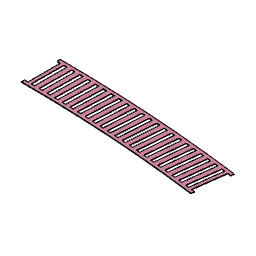
0_15m_Joch_Gebogen_Schablone_v8 (Autodesk Fusion 360 design; units mm, degrees)
Autodesk Fusion 360 part; units mm, degrees
sketch "Skizze4" plane through (0, 0, 0) normal (0, 0, 1) x (1, 0, 0)
  line L0 (0, 0) -> (0, -2516) construction
  circle A0 centre (0, -2516) radius 2516 construction
  line L1 (9.163, 13.0852) -> (9.1, -0.0147)
  line L2 (9.1, -0.0147) -> (15.1, -0.0435)
  line L3 (15.1, -0.0435) -> (15.163, 13.0563)
  line L4 (15.163, 13.0563) -> (9.163, 13.0852)
  line L5 (-3, 13.1) -> (3, 13.1)
  line L6 (3, 13.1) -> (3, 0)
  line L7 (3, 0) -> (-3, 0)
  line L8 (-3, 0) -> (-3, 13.1)
  line L9 (12.163, 13.0708) -> (12.1, -0.0291) construction
  line L10 (23.6378, 12.9913) -> (23.4998, -0.108)
  line L11 (29.4995, -0.1712) -> (29.6374, 12.9281)
  line L12 (26.6376, 12.9597) -> (26.4996, -0.1396) construction
  line L13 (29.6374, 12.9281) -> (23.6378, 12.9913)
  line L14 (23.4998, -0.108) -> (29.4995, -0.1712)
  line L15 (38.1117, 12.8146) -> (37.8988, -0.2837)
  line L16 (58.583, 12.4232) -> (52.5845, 12.5551)
  line L17 (52.2966, -0.5418) -> (58.2951, -0.6736)
  line L18 (52.5845, 12.5551) -> (52.2966, -0.5418)
  line L19 (58.2951, -0.6736) -> (58.583, 12.4232)
  line L20 (55.5837, 12.4891) -> (55.2958, -0.6077) construction
  line L21 (41.1113, 12.7658) -> (40.8984, -0.3324) construction
  line L22 (37.8988, -0.2837) -> (43.898, -0.3812)
  line L23 (43.898, -0.3812) -> (44.111, 12.7171)
  line L24 (44.111, 12.7171) -> (38.1117, 12.8146)
  line L25 (115.8597, -2.6672) -> (116.4473, 10.4196)
  line L26 (101.4731, -2.0453) -> (101.9858, 11.0447)
  line L27 (81.5243, 11.7875) -> (81.0865, -1.3052)
  line L28 (101.9858, 11.0447) -> (95.9904, 11.2795)
  line L29 (67.0555, 12.2127) -> (66.6926, -0.8823)
  line L30 (109.8657, -2.3981) -> (115.8597, -2.6672)
  line L31 (87.5209, 11.587) -> (81.5243, 11.7875)
  line L32 (66.6926, -0.8823) -> (72.6903, -1.0485)
  line L33 (70.0543, 12.1296) -> (69.6914, -0.9654) construction
  line L34 (113.4504, 10.5541) -> (112.8627, -2.5327) construction
  line L35 (81.0865, -1.3052) -> (87.0831, -1.5057)
  line L36 (72.6903, -1.0485) -> (73.0532, 12.0465)
  line L37 (84.5226, 11.6872) -> (84.0848, -1.4055) construction
  line L38 (98.9881, 11.1621) -> (98.4754, -1.9279) construction
  line L39 (95.9904, 11.2795) -> (95.4777, -1.8105)
  line L40 (110.4534, 10.6887) -> (109.8657, -2.3981)
  line L41 (95.4777, -1.8105) -> (101.4731, -2.0453)
  line L42 (116.4473, 10.4196) -> (110.4534, 10.6887)
  line L43 (73.0532, 12.0465) -> (67.0555, 12.2127)
  line L44 (87.0831, -1.5057) -> (87.5209, 11.587)
  line L45 (197.1387, 5.4068) -> (196.1021, -7.6521)
  line L46 (139.368, 9.2589) -> (138.6306, -3.8204)
  line L47 (153.8187, 8.4199) -> (153.0065, -4.6549)
  line L48 (214.5556, 3.9827) -> (213.4443, -9.0701) construction
  line L49 (173.3636, -5.9781) -> (174.2506, 7.0919)
  line L50 (171.2575, 7.295) -> (170.3704, -5.7749) construction
  line L51 (138.6306, -3.8204) -> (144.6211, -4.1581)
  line L52 (153.0065, -4.6549) -> (158.9949, -5.027)
  line L53 (200.1293, 5.1694) -> (199.0927, -7.8895) construction
  line L54 (145.3585, 8.9211) -> (139.368, 9.2589)
  line L55 (211.5664, 4.2372) -> (210.4551, -8.8156)
  line L56 (224.8012, -10.0612) -> (230.7766, -10.6044)
  line L57 (231.9626, 2.4418) -> (225.9872, 2.985)
  line L58 (124.9127, 10.0152) -> (124.2502, -3.0681)
  line L59 (182.7046, 6.4938) -> (181.7427, -6.5709)
  line L60 (167.3773, -5.5718) -> (173.3636, -5.9781)
  line L61 (217.5448, 3.7282) -> (211.5664, 4.2372)
  line L62 (210.4551, -8.8156) -> (216.4335, -9.3246)
  line L63 (228.9749, 2.7134) -> (227.7889, -10.3328) construction
  line L64 (185.6965, 6.2735) -> (184.7346, -6.7911) construction
  line L65 (130.9051, 9.7117) -> (124.9127, 10.0152)
  line L66 (130.2425, -3.3715) -> (130.9051, 9.7117)
  line L67 (202.0833, -8.1269) -> (203.1199, 4.932)
  line L68 (159.8072, 8.0478) -> (153.8187, 8.4199)
  line L69 (158.9949, -5.027) -> (159.8072, 8.0478)
  line L70 (230.7766, -10.6044) -> (231.9626, 2.4418)
  line L71 (168.2644, 7.4981) -> (167.3773, -5.5718)
  line L72 (156.813, 8.2338) -> (156.0007, -4.8409) construction
  line L73 (188.6884, 6.0532) -> (182.7046, 6.4938)
  line L74 (142.3633, 9.09) -> (141.6259, -3.9892) construction
  line L75 (187.7265, -7.0114) -> (188.6884, 6.0532)
  line L76 (127.9089, 9.8634) -> (127.2464, -3.2198) construction
  line L77 (203.1199, 4.932) -> (197.1387, 5.4068)
  line L78 (181.7427, -6.5709) -> (187.7265, -7.0114)
  line L79 (174.2506, 7.0919) -> (168.2644, 7.4981)
  line L80 (196.1021, -7.6521) -> (202.0833, -8.1269)
  line L81 (225.9872, 2.985) -> (224.8012, -10.0612)
  line L82 (144.6211, -4.1581) -> (145.3585, 8.9211)
  line L83 (216.4335, -9.3246) -> (217.5448, 3.7282)
  line L84 (124.2502, -3.0681) -> (130.2425, -3.3715)
  line L85 (0, 13.1) -> (0, 0) construction
  line L86 (243.3867, 1.3617) -> (242.126, -11.6775) construction
  line L87 (275.1684, -1.9121) -> (269.2033, -1.2663)
  line L88 (288.0686, -16.5438) -> (282.1073, -15.8639)
  line L89 (286.5723, -3.1882) -> (285.0879, -16.2038) construction
  line L90 (269.2033, -1.2663) -> (267.7934, -14.2902)
  line L91 (246.3728, 1.073) -> (240.4006, 1.6504)
  line L92 (282.1073, -15.8639) -> (283.5916, -2.8483)
  line L93 (245.1121, -11.9662) -> (246.3728, 1.073)
  line L94 (253.4708, -12.7985) -> (259.4396, -13.4101)
  line L95 (289.553, -3.5281) -> (288.0686, -16.5438)
  line L96 (240.4006, 1.6504) -> (239.1399, -11.3888)
  line L97 (273.7586, -14.936) -> (275.1684, -1.9121)
  line L98 (259.4396, -13.4101) -> (260.7749, -0.3784)
  line L99 (239.1399, -11.3888) -> (245.1121, -11.9662)
  line L100 (254.8061, 0.2332) -> (253.4708, -12.7985)
  line L101 (283.5916, -2.8483) -> (289.553, -3.5281)
  line L102 (260.7749, -0.3784) -> (254.8061, 0.2332)
  line L103 (272.1859, -1.5892) -> (270.776, -14.6131) construction
  line L104 (257.7905, -0.0726) -> (256.4552, -13.1043) construction
  line L105 (267.7934, -14.2902) -> (273.7586, -14.936)
  line L106 (315.3166, -6.6331) -> (313.6833, -19.6309) construction
  line L107 (318.2932, -7.0071) -> (312.34, -6.2591)
  line L108 (322.8097, -20.7928) -> (328.7592, -21.5697)
  line L109 (324.506, -7.8031) -> (322.8097, -20.7928)
  line L110 (316.6599, -20.0049) -> (318.2932, -7.0071)
  line L111 (312.34, -6.2591) -> (310.7067, -19.2569)
  line L112 (303.9281, -5.2265) -> (297.9707, -4.5125)
  line L113 (297.9707, -4.5125) -> (296.4118, -17.5195)
  line L114 (296.4118, -17.5195) -> (302.3692, -18.2334)
  line L115 (300.9494, -4.8695) -> (299.3905, -17.8764) construction
  line L116 (327.4807, -8.1916) -> (325.7844, -21.1813) construction
  line L117 (302.3692, -18.2334) -> (303.9281, -5.2265)
  line L118 (330.4554, -8.58) -> (324.506, -7.8031)
  line L119 (328.7592, -21.5697) -> (330.4554, -8.58)
  line L120 (310.7067, -19.2569) -> (316.6599, -20.0049)
  point P0 (12.1, -0.0291)
  point P1 (26.4996, -0.1396)
  point P2 (55.2958, -0.6077)
  point P3 (40.8984, -0.3324)
  point P4 (112.8627, -2.5327)
  point P5 (98.4754, -1.9279)
  point P6 (84.0848, -1.4055)
  point P7 (69.6914, -0.9654)
  point P8 (170.3704, -5.7749)
  point P9 (156.0007, -4.8409)
  point P10 (199.0927, -7.8895)
  point P11 (184.7346, -6.7911)
  point P12 (213.4443, -9.0701)
  point P13 (227.7889, -10.3328)
  point P14 (141.6259, -3.9892)
  point P15 (127.2464, -3.2198)
  point P16 (256.4552, -13.1043)
  point P17 (242.126, -11.6775)
  point P18 (285.0879, -16.2038)
  point P19 (270.776, -14.6131)
  point P20 (313.6833, -19.6309)
  point P21 (325.7844, -21.1813)
  point P22 (299.3905, -17.8764)
  dimension "d197" = 2516
  dimension "d198" = 6
  dimension "d199" = 13.1
  dimension "d200" = 6
  dimension "d201" = 13.1
  dimension "d202" = 6
  dimension "d203" = 13.1
  dimension "d204" = 6
  dimension "d205" = 13.1
  dimension "d206" = 6
  dimension "d207" = 13.1
  dimension "d208" = 6
  dimension "d209" = 13.1
  dimension "d210" = 6
  dimension "d211" = 13.1
  dimension "d212" = 6
  dimension "d213" = 13.1
  dimension "d214" = 6
  dimension "d215" = 13.1
  dimension "d216" = 6
  dimension "d217" = 13.1
  dimension "d218" = 6
  dimension "d219" = 13.1
  dimension "d220" = 6
  dimension "d221" = 13.1
  dimension "d222" = 6
  dimension "d223" = 13.1
  dimension "d224" = 6
  dimension "d225" = 13.1
  dimension "d226" = 6
  dimension "d227" = 13.1
  dimension "d228" = 6
  dimension "d229" = 13.1
  dimension "d230" = 6
  dimension "d231" = 13.1
  dimension "d232" = 12.1
  dimension "d233" = 14.4
  dimension "d234" = 14.4
  dimension "d235" = 14.4
  dimension "d236" = 14.4
  dimension "d237" = 14.4
  dimension "d238" = 14.4
  dimension "d239" = 14.4
  dimension "d240" = 6
  dimension "d241" = 13.1
  dimension "d242" = 6
  dimension "d243" = 13.1
  dimension "d244" = 6
  dimension "d245" = 13.1
  dimension "d246" = 6
  dimension "d247" = 13.1
  dimension "d248" = 6
  dimension "d249" = 13.1
  dimension "d250" = 6
  dimension "d251" = 13.1
  dimension "d252" = 6
  dimension "d253" = 13.1
  dimension "d254" = 14.4
  dimension "d255" = 14.4
  dimension "d256" = 14.4
  dimension "d257" = 14.4
  dimension "d258" = 14.4
  dimension "d259" = 14.4
  dimension "d260" = 14.4
  dimension "d261" = 14.4
  dimension "d262" = 14.4
  dimension "d263" = 14.4
  dimension "d264" = 14.4
  dimension "d265" = 14.4
  dimension "d266" = 14.4
  dimension "d267" = 14.4
  dimension "d268" = 12.2
  dimension "d269" = 7.4
  constraint coincident L0.start L85.end
  constraint vertical L0
  constraint coincident L0.end A0.centre
  constraint coincident L0.start A0
  constraint perpendicular L1 L2
  constraint parallel L1 L3
  constraint parallel L2 L4
  constraint midpoint L2 P0
  constraint horizontal L5
  constraint vertical L6
  constraint horizontal L7
  constraint vertical L8
  constraint midpoint L0.start L7
  constraint midpoint L4 L9.start
  constraint coincident P0 L9.end
  constraint perpendicular L10 L14
  constraint parallel L10 L11
  constraint parallel L13 L14
  constraint midpoint P1 L14
  constraint midpoint L12.start L13
  constraint coincident P1 L12.end
  constraint perpendicular L15 L22
  constraint parallel L15 L23
  constraint parallel L22 L24
  constraint midpoint P3 L22
  constraint midpoint L21.start L24
  constraint coincident P3 L21.end
  constraint perpendicular L17 L18
  constraint parallel L18 L19
  constraint parallel L16 L17
  constraint midpoint P2 L17
  constraint midpoint L20.start L16
  constraint coincident P2 L20.end
  constraint perpendicular L29 L32
  constraint parallel L29 L36
  constraint parallel L32 L43
  constraint midpoint P7 L32
  constraint midpoint L33.start L43
  constraint coincident P7 L33.end
  constraint perpendicular L27 L35
  constraint parallel L27 L44
  constraint parallel L31 L35
  constraint midpoint P6 L35
  constraint midpoint L37.start L31
  constraint coincident P6 L37.end
  constraint perpendicular L39 L41
  constraint parallel L26 L39
  constraint parallel L28 L41
  constraint midpoint P5 L41
  constraint midpoint L38.start L28
  constraint coincident P5 L38.end
  constraint perpendicular L30 L40
  constraint parallel L25 L40
  constraint parallel L30 L42
  constraint midpoint P4 L30
  constraint midpoint L34.start L42
  constraint coincident P4 L34.end
  constraint perpendicular L58 L84
  constraint parallel L58 L66
  constraint parallel L65 L84
  constraint midpoint P15 L84
  constraint midpoint L76.start L65
  constraint coincident P15 L76.end
  constraint perpendicular L46 L51
  constraint parallel L46 L82
  constraint parallel L51 L54
  constraint midpoint P14 L51
  constraint midpoint L74.start L54
  constraint coincident P14 L74.end
  constraint perpendicular L47 L52
  constraint parallel L47 L69
  constraint parallel L52 L68
  constraint midpoint P9 L52
  constraint midpoint L72.start L68
  constraint coincident P9 L72.end
  constraint perpendicular L60 L71
  constraint parallel L49 L71
  constraint parallel L60 L79
  constraint midpoint P8 L60
  constraint midpoint L50.start L79
  constraint coincident P8 L50.end
  constraint perpendicular L59 L78
  constraint parallel L59 L75
  constraint parallel L73 L78
  constraint midpoint P11 L78
  constraint midpoint L64.start L73
  constraint coincident P11 L64.end
  constraint perpendicular L45 L80
  constraint parallel L45 L67
  constraint parallel L77 L80
  constraint midpoint P10 L80
  constraint midpoint L53.start L77
  constraint coincident P10 L53.end
  constraint perpendicular L55 L62
  constraint parallel L55 L83
  constraint parallel L61 L62
  constraint midpoint P12 L62
  constraint midpoint L48.start L61
  constraint coincident P12 L48.end
  constraint perpendicular L56 L81
  constraint parallel L70 L81
  constraint parallel L56 L57
  constraint midpoint P13 L56
  constraint midpoint L63.start L57
  constraint coincident P13 L63.end
  constraint midpoint L5 L85.start
  constraint coincident A0 P0
  constraint coincident A0 P1
  constraint coincident A0 P3
  constraint coincident A0 P2
  constraint coincident A0 P7
  constraint coincident A0 P6
  constraint coincident A0 P5
  constraint coincident A0 P4
  constraint tangent A0 L2
  constraint tangent A0 L14
  constraint tangent A0 L22
  constraint tangent A0 L17
  constraint tangent A0 L32
  constraint tangent A0 L35
  constraint tangent A0 L41
  constraint tangent A0 L30
  constraint coincident A0 P15
  constraint coincident A0 P14
  constraint coincident A0 P9
  constraint coincident A0 P8
  constraint perpendicular L96 L99
  constraint parallel L93 L96
  constraint parallel L91 L99
  constraint midpoint P17 L99
  constraint midpoint L86.start L91
  constraint coincident P17 L86.end
  constraint perpendicular L94 L100
  constraint parallel L98 L100
  constraint parallel L94 L102
  constraint midpoint P16 L94
  constraint midpoint L104.start L102
  constraint coincident P16 L104.end
  constraint perpendicular L90 L105
  constraint parallel L90 L97
  constraint parallel L87 L105
  constraint midpoint P19 L105
  constraint midpoint L103.start L87
  constraint coincident P19 L103.end
  constraint perpendicular L88 L95
  constraint parallel L92 L95
  constraint parallel L88 L101
  constraint midpoint P18 L88
  constraint midpoint L89.start L101
  constraint coincident P18 L89.end
  constraint perpendicular L113 L114
  constraint parallel L113 L117
  constraint parallel L112 L114
  constraint midpoint P22 L114
  constraint midpoint L115.start L112
  constraint coincident P22 L115.end
  constraint perpendicular L111 L120
  constraint parallel L110 L111
  constraint parallel L107 L120
  constraint midpoint P20 L120
  constraint midpoint L106.start L107
  constraint coincident P20 L106.end
  constraint perpendicular L108 L109
  constraint parallel L109 L119
  constraint parallel L108 L118
  constraint midpoint P21 L108
  constraint midpoint L116.start L118
  constraint coincident P21 L116.end
  constraint coincident A0 P11
  constraint coincident A0 P10
  constraint coincident A0 P12
  constraint coincident A0 P13
  constraint tangent A0 L84
  constraint tangent A0 L51
  constraint tangent A0 L52
  constraint tangent A0 L60
  constraint tangent A0 L78
  constraint tangent A0 L80
  constraint tangent A0 L62
  constraint tangent A0 L56
  constraint coincident A0 P17
  constraint coincident A0 P16
  constraint coincident A0 P19
  constraint coincident A0 P18
  constraint coincident A0 P22
  constraint coincident A0 P20
  constraint coincident A0 P21
  constraint tangent A0 L99
  constraint tangent A0 L94
  constraint tangent A0 L105
  constraint tangent A0 L88
  constraint tangent A0 L114
  constraint tangent A0 L120
  constraint tangent A0 L108
  measures "d197" distance of L0.start L0.end
  measures "d198" distance of L1 L3
  measures "d199" distance of L2 L4
  measures "d200" distance of L6 L8
  measures "d201" distance of L5 L7
  measures "d202" distance of L10 L11
  measures "d203" distance of L13 L14
  measures "d204" distance of L15 L23
  measures "d205" distance of L22 L24
  measures "d206" distance of L18 L19
  measures "d207" distance of L16 L17
  measures "d208" distance of L29 L36
  measures "d209" distance of L32 L43
  measures "d210" distance of L27 L44
  measures "d211" distance of L31 L35
  measures "d212" distance of L26 L39
  measures "d213" distance of L28 L41
  measures "d214" distance of L25 L40
  measures "d215" distance of L30 L42
  measures "d216" distance of L58 L66
  measures "d217" distance of L65 L84
  measures "d218" distance of L46 L82
  measures "d219" distance of L51 L54
  measures "d220" distance of L47 L69
  measures "d221" distance of L52 L68
  measures "d222" distance of L49 L71
  measures "d223" distance of L60 L79
  measures "d224" distance of L59 L75
  measures "d225" distance of L73 L78
  measures "d226" distance of L45 L67
  measures "d227" distance of L77 L80
  measures "d228" distance of L55 L83
  measures "d229" distance of L61 L62
  measures "d230" distance of L70 L81
  measures "d231" distance of L56 L57
  measures "d232" distance of P0 L85
  measures "d233" distance of L9 P1
  measures "d234" distance of L12 P3
  measures "d235" distance of P2 L21
  measures "d236" distance of L20 P7
  measures "d237" distance of P6 L33
  measures "d238" distance of P5 L37
  measures "d239" distance of P4 L38
  measures "d240" distance of L93 L96
  measures "d241" distance of L91 L99
  measures "d242" distance of L98 L100
  measures "d243" distance of L94 L102
  measures "d244" distance of L90 L97
  measures "d245" distance of L87 L105
  measures "d246" distance of L92 L95
  measures "d247" distance of L88 L101
  measures "d248" distance of L113 L117
  measures "d249" distance of L112 L114
  measures "d250" distance of L110 L111
  measures "d251" distance of L107 L120
  measures "d252" distance of L109 L119
  measures "d253" distance of L108 L118
  measures "d254" distance of L34 P15
  measures "d255" distance of P14 L76
  measures "d256" distance of P9 L74
  measures "d257" distance of P8 L72
  measures "d258" distance of P11 L50
  measures "d259" distance of P10 L64
  measures "d260" distance of P12 L53
  measures "d261" distance of P13 L48
  measures "d262" distance of L63 P17
  measures "d263" distance of P16 L86
  measures "d264" distance of P19 L104
  measures "d265" distance of P18 L103
  measures "d266" distance of L89 P22
  measures "d267" distance of P20 L115
  measures "d268" distance of P21 L106
extrude "Extrusion1" add sketch "Skizze4" along normal blind 3 makes body 1 at (27.5456, 4.2163, 0) makes body 2 at (83.2313, 2.9922, 0) makes body 3 at (140.8732, 0.4268, 0) makes body 4 at (198.4414, -3.4574, 0) makes body 5 at (258.3402, -4.5184, 0) makes body 6 at (313.2355, -15.1736, 0) makes body 7 at (298.9172, -13.4218, 0) makes body 8 at (243.5416, -7.4274, 0) makes body 9 at (184.0579, -2.3628, 0) makes body 10 at (126.4685, 1.1919, 0) makes body 11 at (68.8128, 3.4273, 0) makes body 12 at (13.121, 4.3327, 0) makes body 13 at (39.9695, 4.0499, 0) makes body 14 at (97.647, 2.4746, 0) makes body 15 at (155.2734, -0.4207, 0) makes body 16 at (212.8183, -4.6343, 0) makes body 17 at (270.2518, -10.1642, 0) makes body 18 at (327.9069, -12.6509, 0) makes body 19 at (287.0711, -7.6401, 0) makes body 20 at (229.1801, -6.0746, 0) makes body 21 at (169.6684, -1.3506, 0) makes body 22 at (112.2555, 6.2367, 0) makes body 23 at (54.392, 3.7799, 0) makes body 24 at (-1, 4.3667, 0)
move_face "Flächen versetzen1" offset 45.1 24 faces at (300.3834, -17.9954, 2) (241.1307, -11.5813, 1) (183.7373, -6.7177, 1) (128.2451, -3.2704, 2) (83.0853, -1.372, 1) (25.4997, -0.129, 1) (255.4604, -13.0024, 1) (314.6755, -19.7556, 2) (198.0958, -7.8104, 1) (140.6274, -3.9329, 1) (68.6918, -0.9377, 1) (13.1, -0.0339, 2) (39.8985, -0.3162, 1) (97.4761, -1.8887, 2) (155.0026, -4.7789, 1) (212.4479, -8.9853, 1) (269.7818, -14.5055, 1) (324.7929, -21.0518, 1) (286.0815, -16.3171, 1) (226.793, -10.2422, 1) (169.3727, -5.7072, 1) (111.8637, -2.4878, 1) (54.2961, -0.5857, 1) (1, 0, 1) on bodies 1 2 3 4 5 6 7 8 9 10 11 12 13 14 15 16 17 18 19 20 21 22 23 24
sketch "Skizze5" plane through (0, 0, 0) normal (0, 0, 1) x (1, 0, 0)
  line L0 (-3, 13.1) -> (-3, -45.1)
  line L1 (322.9194, -66.29) -> (330.4554, -8.58)
  line L2 (-3, 13.1) -> (-3, 18.7667)
  line L3 (-3, -45.1) -> (-3, -50.7667)
  line L4 (330.4554, -8.58) -> (331.1892, -2.9611)
  line L5 (322.9194, -66.29) -> (322.1856, -71.909)
  arc A0 (331.1892, -2.9611) -> (-3, 18.7667) centre (-3, -2562.142) ccw
  arc A1 (322.1856, -71.909) -> (-3, -50.7667) centre (-3, -2562.142) ccw
  line L6 (-3, 18.7667) -> (-30, 18.7667)
  line L7 (-3, -50.7667) -> (-34, -50.7667)
  dimension "d273" = 5.6667
  dimension "d274" = 5.6667
  dimension "d275" = 5.6667
  dimension "d276" = 5.6667
  constraint coincident L0.start L2.start
  constraint coincident L0.end L3.start
  constraint coincident L1.end L4.start
  constraint coincident L1.start L5.start
  constraint parallel L0 L2
  constraint parallel L0 L3
  constraint parallel L1 L5
  constraint parallel L1 L4
  constraint perpendicular L2 L6
  constraint tangent A0 L6
  constraint perpendicular L3 L7
  constraint tangent A1 L7
  measures "d273" distance of L0.start L2.end
  measures "d274" distance of L0.end L3.end
  measures "d275" distance of L1.end L4.end
  measures "d276" distance of L1.start L5.end
extrude "Extrusion2" add sketch "Skizze5" along normal blind 1 separate body makes body 25
combine "Kombinieren1" operation cut target body 25 tool bodies 18 6 7 19 17 5 8 20 16 4 9 21 15 3 10 22 14 2 11 23 13 1 12 24 keep tools
sketch "Skizze8" plane through (0, 0, 1) normal (0, 0, 1) x (-1, 0, 0)
  line L0 (-3, 45.1) -> (3, 45.1)
  line L1 (3, 45.1) -> (3, 50.7667)
  arc A0 (-322.1856, 71.909) -> (3, 50.7667) centre (3, 2562.142) ccw
  line L2 (-322.1856, 71.909) -> (-322.9194, 66.29)
  line L3 (-322.9194, 66.29) -> (-316.9699, 65.5131)
  line L4 (-316.9699, 65.5131) -> (-324.506, 7.8031)
  line L5 (-324.506, 7.8031) -> (-330.4554, 8.58)
  line L6 (-330.4554, 8.58) -> (-331.1892, 2.9611)
  arc A1 (-331.1892, 2.9611) -> (3, -18.7667) centre (3, 2562.142) ccw
  line L7 (3, -18.7667) -> (3, -13.1)
  line L8 (3, -13.1) -> (-3, -13.1)
  line L9 (-3, -13.1) -> (-3, 45.1)
  line L10 (-15.163, -13.0563) -> (-14.8831, 45.143)
  line L11 (-14.8831, 45.143) -> (-8.8831, 45.1141)
  line L12 (-8.8831, 45.1141) -> (-9.163, -13.0852)
  line L13 (-9.163, -13.0852) -> (-15.163, -13.0563)
  line L14 (-23.0248, 45.2055) -> (-23.6378, -12.9913)
  line L15 (-23.6378, -12.9913) -> (-29.6374, -12.9281)
  line L16 (-29.6374, -12.9281) -> (-29.0245, 45.2687)
  line L17 (-29.0245, 45.2687) -> (-23.0248, 45.2055)
  line L18 (-44.111, -12.7171) -> (-43.1649, 45.4752)
  line L19 (-43.1649, 45.4752) -> (-37.1657, 45.3777)
  line L20 (-37.1657, 45.3777) -> (-38.1117, -12.8146)
  line L21 (-38.1117, -12.8146) -> (-44.111, -12.7171)
  line L22 (-57.3039, 45.7628) -> (-51.3054, 45.6309)
  line L23 (-51.3054, 45.6309) -> (-52.5845, -12.5551)
  line L24 (-52.5845, -12.5551) -> (-58.583, -12.4232)
  line L25 (-58.583, -12.4232) -> (-57.3039, 45.7628)
  line L26 (-73.0532, -12.0465) -> (-71.441, 46.1312)
  line L27 (-71.441, 46.1312) -> (-65.4433, 45.965)
  line L28 (-65.4433, 45.965) -> (-67.0555, -12.2127)
  line L29 (-67.0555, -12.2127) -> (-73.0532, -12.0465)
  line L30 (-85.5758, 46.5805) -> (-79.5792, 46.38)
  line L31 (-79.5792, 46.38) -> (-81.5243, -11.7875)
  line L32 (-81.5243, -11.7875) -> (-87.5209, -11.587)
  line L33 (-87.5209, -11.587) -> (-85.5758, 46.5805)
  line L34 (-93.7124, 46.8759) -> (-95.9904, -11.2795)
  line L35 (-95.9904, -11.2795) -> (-101.9858, -11.0447)
  line L36 (-101.9858, -11.0447) -> (-99.7078, 47.1107)
  line L37 (-99.7078, 47.1107) -> (-93.7124, 46.8759)
  line L38 (-116.4473, -10.4196) -> (-113.8366, 47.7218)
  line L39 (-113.8366, 47.7218) -> (-107.8426, 47.4527)
  line L40 (-107.8426, 47.4527) -> (-110.4534, -10.6887)
  line L41 (-110.4534, -10.6887) -> (-116.4473, -10.4196)
  line L42 (-121.9693, 48.1104) -> (-124.9127, -10.0152)
  line L43 (-124.9127, -10.0152) -> (-130.9051, -9.7117)
  line L44 (-130.9051, -9.7117) -> (-127.9616, 48.4138)
  line L45 (-127.9616, 48.4138) -> (-121.9693, 48.1104)
  line L46 (-142.0824, 49.1866) -> (-136.0919, 48.8488)
  line L47 (-136.0919, 48.8488) -> (-139.368, -9.2589)
  line L48 (-139.368, -9.2589) -> (-145.3585, -8.9211)
  line L49 (-145.3585, -8.9211) -> (-142.0824, 49.1866)
  line L50 (-156.1986, 50.0402) -> (-150.2101, 49.6682)
  line L51 (-150.2101, 49.6682) -> (-153.8187, -8.4199)
  line L52 (-153.8187, -8.4199) -> (-159.8072, -8.0478)
  line L53 (-159.8072, -8.0478) -> (-156.1986, 50.0402)
  line L54 (-174.2506, -7.0919) -> (-170.3096, 50.9746)
  line L55 (-170.3096, 50.9746) -> (-164.3234, 50.5683)
  line L56 (-164.3234, 50.5683) -> (-168.2644, -7.4981)
  line L57 (-168.2644, -7.4981) -> (-174.2506, -7.0919)
  line L58 (-178.4313, 51.5491) -> (-182.7046, -6.4938)
  line L59 (-182.7046, -6.4938) -> (-188.6884, -6.0532)
  line L60 (-188.6884, -6.0532) -> (-184.4151, 51.9897)
  line L61 (-184.4151, 51.9897) -> (-178.4313, 51.5491)
  line L62 (-192.5333, 52.6107) -> (-197.1387, -5.4068)
  line L63 (-197.1387, -5.4068) -> (-203.1199, -4.932)
  line L64 (-203.1199, -4.932) -> (-198.5145, 53.0855)
  line L65 (-198.5145, 53.0855) -> (-192.5333, 52.6107)
  line L66 (-212.6074, 54.262) -> (-206.629, 53.753)
  line L67 (-206.629, 53.753) -> (-211.5664, -4.2372)
  line L68 (-211.5664, -4.2372) -> (-217.5448, -3.7282)
  line L69 (-217.5448, -3.7282) -> (-212.6074, 54.262)
  line L70 (-225.9872, -2.985) -> (-231.9626, -2.4418)
  line L71 (-231.9626, -2.4418) -> (-226.6934, 55.5192)
  line L72 (-226.6934, 55.5192) -> (-220.718, 54.9759)
  line L73 (-220.718, 54.9759) -> (-225.9872, -2.985)
  line L74 (-234.7997, 56.2795) -> (-240.4006, -1.6504)
  line L75 (-240.4006, -1.6504) -> (-246.3728, -1.073)
  line L76 (-246.3728, -1.073) -> (-240.7719, 56.8569)
  line L77 (-240.7719, 56.8569) -> (-234.7997, 56.2795)
  line L78 (-260.7749, 0.3784) -> (-254.8425, 58.2752)
  line L79 (-254.8425, 58.2752) -> (-248.8738, 57.6636)
  line L80 (-248.8738, 57.6636) -> (-254.8061, -0.2332)
  line L81 (-254.8061, -0.2332) -> (-260.7749, 0.3784)
  line L82 (-262.9397, 59.1283) -> (-269.2033, 1.2663)
  line L83 (-269.2033, 1.2663) -> (-275.1684, 1.9121)
  line L84 (-275.1684, 1.9121) -> (-268.9048, 59.774)
  line L85 (-268.9048, 59.774) -> (-262.9397, 59.1283)
  line L86 (-283.5916, 2.8483) -> (-289.553, 3.5281)
  line L87 (-289.553, 3.5281) -> (-282.9583, 61.3533)
  line L88 (-282.9583, 61.3533) -> (-276.9969, 60.6734)
  line L89 (-276.9969, 60.6734) -> (-283.5916, 2.8483)
  line L90 (-297.0025, 63.013) -> (-291.0451, 62.299)
  line L91 (-291.0451, 62.299) -> (-297.9707, 4.5125)
  line L92 (-297.9707, 4.5125) -> (-303.9281, 5.2265)
  line L93 (-303.9281, 5.2265) -> (-297.0025, 63.013)
  line L94 (-305.0838, 64.005) -> (-312.34, 6.2591)
  line L95 (-312.34, 6.2591) -> (-318.2932, 7.0071)
  line L96 (-318.2932, 7.0071) -> (-311.037, 64.753)
  line L97 (-311.037, 64.753) -> (-305.0838, 64.005)
  line L98 (-3, -13.1) -> (-3, 45.1)
  line L99 (-8.8831, 45.1141) -> (-9.163, -13.0852)
  line L100 (-15.163, -13.0563) -> (-14.8831, 45.143)
  line L101 (-23.0248, 45.2055) -> (-23.6378, -12.9913)
  line L102 (-29.6374, -12.9281) -> (-29.0245, 45.2687)
  line L103 (-316.9699, 65.5131) -> (-324.506, 7.8031)
  line L104 (-318.2932, 7.0071) -> (-311.037, 64.753)
  line L105 (-305.0838, 64.005) -> (-312.34, 6.2591)
  line L106 (-303.9281, 5.2265) -> (-297.0025, 63.013)
  line L107 (-291.0451, 62.299) -> (-297.9707, 4.5125)
  line L108 (-3, 16) -> (7, 16)
  arc A2 (-320.7379, 36.6581) -> (-3, 16) centre (-3, 2469.858) ccw
  circle A3 centre (-3, 16) radius 1
  circle A4 centre (-9.0231, 16.0145) radius 1
  circle A5 centre (-15.023, 16.0433) radius 1
  circle A6 centre (-23.3313, 16.1071) radius 1
  point P0 (-3, 16)
  point P1 (-9.0231, 16.0145)
  point P2 (-15.023, 16.0433)
  point P3 (-23.3313, 16.1071)
  dimension "d502" = 10
  dimension "d503" = 2
  dimension "d504" = 2
  dimension "d506" = 2
  dimension "d507" = 2
  constraint midpoint L98 P0
  constraint perpendicular L98 L108
  constraint tangent L108 A2
  constraint midpoint L103 A2.start
  constraint coincident P0 L108.start
  constraint midpoint L12 P1
  constraint midpoint L10 P2
  constraint midpoint L14 P3
  constraint coincident P1 A4.centre
  constraint coincident P2 A5.centre
  constraint coincident P3 A6.centre
  measures "d502" distance of P0 L108.end
  measures "d503" diameter of A3
  measures "d504" diameter of A4
  measures "d506" diameter of A5
  measures "d507" diameter of A6
hidden bodies 1 2 3 4 5 6 7 8 9 10 11 12 13 14 15 16 17 18 19 20 21 22 23 24
equation "Schwellen_Länge = 58 mm + 0.2 mm"
equation "Schwellen_Breite = 5.8 mm + 0.2 mm"
equation "Bogen_Radius = 2500 mm"
equation "Spurweite = 32 mm"
equation "d197 = Bogen_Radius + ( Spurweite / 2 )"
equation "d198 = Schwellen_Breite"
equation "d199 = ( Schwellen_Länge / 2 ) - ( Spurweite / 2 )"
equation "d200 = Schwellen_Breite"
equation "d201 = ( Schwellen_Länge / 2 ) - ( Spurweite / 2 )"
equation "d202 = Schwellen_Breite"
equation "d203 = ( Schwellen_Länge / 2 ) - ( Spurweite / 2 )"
equation "d204 = Schwellen_Breite"
equation "d205 = ( Schwellen_Länge / 2 ) - ( Spurweite / 2 )"
equation "d206 = Schwellen_Breite"
equation "d207 = ( Schwellen_Länge / 2 ) - ( Spurweite / 2 )"
equation "d208 = Schwellen_Breite"
equation "d209 = ( Schwellen_Länge / 2 ) - ( Spurweite / 2 )"
equation "d210 = Schwellen_Breite"
equation "d211 = ( Schwellen_Länge / 2 ) - ( Spurweite / 2 )"
equation "d212 = Schwellen_Breite"
equation "d213 = ( Schwellen_Länge / 2 ) - ( Spurweite / 2 )"
equation "d214 = Schwellen_Breite"
equation "d215 = ( Schwellen_Länge / 2 ) - ( Spurweite / 2 )"
equation "d216 = Schwellen_Breite"
equation "d217 = ( Schwellen_Länge / 2 ) - ( Spurweite / 2 )"
equation "d218 = Schwellen_Breite"
equation "d219 = ( Schwellen_Länge / 2 ) - ( Spurweite / 2 )"
equation "d220 = Schwellen_Breite"
equation "d221 = ( Schwellen_Länge / 2 ) - ( Spurweite / 2 )"
equation "d222 = Schwellen_Breite"
equation "d223 = ( Schwellen_Länge / 2 ) - ( Spurweite / 2 )"
equation "d224 = Schwellen_Breite"
equation "d225 = ( Schwellen_Länge / 2 ) - ( Spurweite / 2 )"
equation "d226 = Schwellen_Breite"
equation "d227 = ( Schwellen_Länge / 2 ) - ( Spurweite / 2 )"
equation "d228 = Schwellen_Breite"
equation "d229 = ( Schwellen_Länge / 2 ) - ( Spurweite / 2 )"
equation "d230 = Schwellen_Breite"
equation "d231 = ( Schwellen_Länge / 2 ) - ( Spurweite / 2 )"
equation "d232 = Schwellen_Abstand_Anfang"
equation "d233 = Schwellen_Abstand_Mitte"
equation "d234 = Schwellen_Abstand_Mitte"
equation "d235 = Schwellen_Abstand_Mitte"
equation "d236 = Schwellen_Abstand_Mitte"
equation "d237 = Schwellen_Abstand_Mitte"
equation "d238 = Schwellen_Abstand_Mitte"
equation "d239 = Schwellen_Abstand_Mitte"
equation "d240 = Schwellen_Breite"
equation "d241 = ( Schwellen_Länge / 2 ) - ( Spurweite / 2 )"
equation "d242 = Schwellen_Breite"
equation "d243 = ( Schwellen_Länge / 2 ) - ( Spurweite / 2 )"
equation "d244 = Schwellen_Breite"
equation "d245 = ( Schwellen_Länge / 2 ) - ( Spurweite / 2 )"
equation "d246 = Schwellen_Breite"
equation "d247 = ( Schwellen_Länge / 2 ) - ( Spurweite / 2 )"
equation "d248 = Schwellen_Breite"
equation "d249 = ( Schwellen_Länge / 2 ) - ( Spurweite / 2 )"
equation "d250 = Schwellen_Breite"
equation "d251 = ( Schwellen_Länge / 2 ) - ( Spurweite / 2 )"
equation "d252 = Schwellen_Breite"
equation "d253 = ( Schwellen_Länge / 2 ) - ( Spurweite / 2 )"
equation "d254 = Schwellen_Abstand_Mitte"
equation "d255 = Schwellen_Abstand_Mitte"
equation "d256 = Schwellen_Abstand_Mitte"
equation "d257 = Schwellen_Abstand_Mitte"
equation "d258 = Schwellen_Abstand_Mitte"
equation "d259 = Schwellen_Abstand_Mitte"
equation "d260 = Schwellen_Abstand_Mitte"
equation "d261 = Schwellen_Abstand_Mitte"
equation "d262 = Schwellen_Abstand_Mitte"
equation "d263 = Schwellen_Abstand_Mitte"
equation "d264 = Schwellen_Abstand_Mitte"
equation "d265 = Schwellen_Abstand_Mitte"
equation "d266 = Schwellen_Abstand_Mitte"
equation "d267 = Schwellen_Abstand_Mitte"
equation "d268 = Schwellen_Abstand_Ende"
equation "d272 = ( Schwellen_Länge / 2 ) + ( Spurweite / 2 )"
equation "d273 = ( Trassenbrett_Breite / Schwellen_Breite / 2 ) * 1 mm"
equation "d274 = d273"
equation "d275 = d273"
equation "d276 = d273"
equation "Schwellen_Abstand_Anfang = 12.1 mm"
equation "Schwellen_Abstand_Mitte = 14.4 mm"
equation "Schwellen_Abstand_Ende = 12.2 mm"
equation "Trassenbrett_Breite = 68 mm"
equation "d503 = Trennstelle_Durchmesser"
equation "d504 = Trennstelle_Durchmesser"
equation "Trennstelle_Durchmesser = 2 mm"
equation "d506 = Trennstelle_Durchmesser"
equation "d507 = Trennstelle_Durchmesser"
named bodies: "Schablone"
